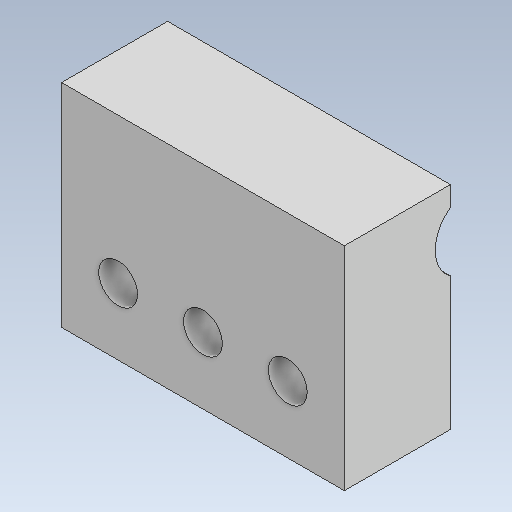
# Autodesk Inventor part: 0008-10-011 Fixare AxaX Mijloc
Saved by Autodesk Inventor 2020 (Build 240168000, 168)
## iProperties
Created: 2021-02-27
Part Number: 0008-10-011 Fixare AxaX Mijloc
Material: Generic
Document SubType Name: Modeling
Designer: Iulian Bors
Density: 1 g/cm^3
Appearance: Default
Description: Fixare Axa mijloc
Mass: 16.4264 g
Surface Area: 51.6587 cm^2
Volume: 16.4264 cm^3
Author: Iulian Bors
Subject: 011
Autodesk Inventor part; units mm, degrees
ref_plane "YZ Plane" through (0, 0, 0) normal (1, 0, 0) x (0, 1, 0)
ref_plane "XZ Plane" through (0, 0, 0) normal (0, 1, 0) x (-1, 0, 0)
ref_plane "XY Plane" through (0, 0, 0) normal (0, 0, 1) x (1, 0, 0)
sketch "Sketch1" plane through (0, 0, 0) normal (0, 0, 1) x (1, 0, 0)
  line L0 (-20, 15) -> (20, 15)
  line L1 (20, 15) -> (20, -15)
  line L2 (20, -15) -> (-20, -15)
  line L3 (-20, -15) -> (-20, 15)
  point P0 (0, 0)
  point P1 (-20, 0)
  point P2 (0, 15)
  dimension "d0" = 30
  dimension "d1" = 40
  constraints: 8 end point, 2 midpoint, 2 parallel, 1 horizontal, 1 horizontal alignment, 1 perpendicular, 1 vertical alignment
  measures "d0" distance of L2.end L0.start
  measures "d1" distance of L0.start L0.end
extrude "Extrusion1" add sketch "Sketch1" along normal blind 15
sketch "Sketch2" plane through (-20, -15, 0) normal (-1, 0, 0) x (0, 0, 1)
  circle A0 centre (-3, 23) radius 5.15
  line L0 (0, 30) -> (0, 0) projected
  line L1 (0, 0) -> (15, 0) projected
  point P0 (0, 15)
  point P1 (0, 15)
  dimension "d5" = 10.3
  dimension "d17" = 23
  dimension "d18" = 3
  constraints: 1 centre point, 1 midpoint
  measures "d5" diameter of A0
  measures "d17" distance from line of A0.centre L1
  measures "d18" distance from line of L0 A0.centre
extrude "Extrusion2" cut sketch "Sketch2" against normal through all
sketch "Sketch3" plane through (0, 0, 0) normal (0, 0, -1) x (-1, 0, 0)
  line L0 (-20, -15) -> (-20, 15) projected
  line L1 (-20, -15) -> (-20, 3.814) projected
  line L2 (20, -15) -> (-20, -15) projected
  line L3 (-20, 15) -> (20, 15) projected
  line L4 (20, 3.814) -> (20, -15) projected
  point P0 (0, 0)
  point P1 (-12, -5.593)
  point P2 (-20, 0)
  point P3 (-20, 12.186)
  point P4 (-20, -5.593)
  point P5 (0, 15)
  point P6 (0, -5.593)
  point P7 (12, -5.593)
  dimension "d19" = 8
  dimension "d20" = 8
  constraints: 3 horizontal alignment, 3 midpoint, 1 vertical alignment
  measures "d19" distance of point (-20, -5.593) point (-12, -5.593)
  measures "d20" distance from line of L4 point (12, -5.593)
hole "Hole1" at (12, -5.593, 0) at (0, -5.593, 0) at (-12, -5.593, 0) direction (0, 0, 1) diameter 5.5 end through all
equation "\"d20\" = d19"
body "Solid1"
